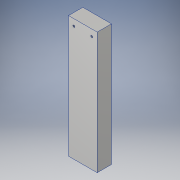
# Autodesk Inventor part: HingeBrace
Saved by Autodesk Inventor 2019 (Build 230136000, 136)
## iProperties
Created: 2019-03-12
Part Number: HingeBrace
Material: Aluminum 6061
Document SubType Name: Modeling
Designer: User
Density: 2.7 g/cm^3
Appearance: Aluminum - Flat
Author: User
Autodesk Inventor part; units mm, degrees
ref_plane "YZ Plane" through (0, 0, 0) normal (1, 0, 0) x (0, 1, 0)
ref_plane "XZ Plane" through (0, 0, 0) normal (0, 1, 0) x (-1, 0, 0)
ref_plane "XY Plane" through (0, 0, 0) normal (0, 0, 1) x (1, 0, 0)
sketch "Sketch1" plane through (0, 0, 0) normal (0, 0, 1) x (1, 0, 0)
  line L0 (0, 0) -> (25.4, 0)
  line L1 (25.4, 0) -> (25.4, 107.95)
  line L2 (25.4, 107.95) -> (0, 107.95)
  line L3 (0, 107.95) -> (0, 0)
  dimension "d0" = 25.4
  dimension "d1" = 107.95
  constraints: 8 end point, 2 parallel, 1 horizontal, 1 perpendicular
  measures "d0" distance of L2.end L1.end
  measures "d1" distance of L1.end L0.end
extrude "Extrusion1" add sketch "Sketch1" along normal blind 12.7
sketch "Sketch2" plane through (0, 0, 12.7) normal (0, 0, 1) x (1, 0, 0)
  line L0 (25.4, 107.95) -> (0, 107.95) projected
  line L1 (0, 107.95) -> (0, 0) projected
  point P0 (4.7625, 102.1588)
  point P1 (20.6375, 102.1588)
  dimension "d4" = 15.875
  dimension "d5" = 5.7912
  dimension "d6" = 5.7912
  dimension "d7" = 25.4
  dimension "d8" = 4.7625
  measures "d4" distance of point (20.637, 102.159) point (4.762, 102.159)
  measures "d5" distance from line of L0 point (4.762, 102.159)
  measures "d6" distance from line of L0 point (20.637, 102.159)
  measures "d7" distance of L0.start L0.end
  measures "d8" distance from line of L1 point (4.762, 102.159)
hole "Hole1" at (20.6375, 102.1588, 12.7) at (4.7625, 102.1588, 12.7) direction (0, 0, -1) diameter 1.7018 end through all
equation "\"d6\" = d5"
equation "\"d8\" = -0.5 * d4 + 0.5 * d7"
body "Solid1"
